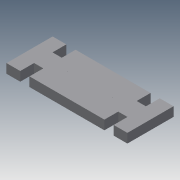
# Autodesk Inventor part: prepazka-sablona
Saved by Autodesk Inventor 2013 (Build 170138000, 138)
## iProperties
Created: 2012-08-25
Part Number: prepazka-sablona
Material: Generic
Document SubType Name: Modeling
Designer: idle-rug
Density: 1 g/cm^3
Author: idle-rug
Autodesk Inventor part; units mm, degrees
ref_plane "YZ Plane" through (0, 0, 0) normal (1, 0, 0) x (0, 1, 0)
ref_plane "XZ Plane" through (0, 0, 0) normal (0, 1, 0) x (-1, 0, 0)
ref_plane "XY Plane" through (0, 0, 0) normal (0, 0, 1) x (1, 0, 0)
sketch "Sketch1" plane through (0, 0, 0) normal (0, 0, 1) x (1, 0, 0)
  line L0 (65.5, 25) -> (-65.5, 25)
  line L1 (-65.5, 25) -> (-65.5, -25)
  line L2 (-65.5, -25) -> (65.5, -25)
  line L3 (65.5, -25) -> (65.5, 25)
  line L4 (-40.6, 25) -> (-40.6, 10)
  line L5 (-40.6, 10) -> (-50.6, 10)
  line L6 (-50.6, 10) -> (-50.6, 25)
  line L7 (-40.6, -25) -> (-40.6, -10)
  line L8 (-40.6, -10) -> (-50.6, -10)
  line L9 (-50.6, -10) -> (-50.6, -25)
  line L10 (40.6, 25) -> (40.6, 10)
  line L11 (40.6, 10) -> (50.6, 10)
  line L12 (50.6, 10) -> (50.6, 25)
  line L13 (40.6, -25) -> (40.6, -10)
  line L14 (40.6, -10) -> (50.6, -10)
  line L15 (50.6, -10) -> (50.6, -25)
  circle A0 centre (-24.1, 0) radius 0.2
  circle A1 centre (24.1, 0) radius 0.2
  point P0 (0, 0)
  point P1 (0, 0)
  dimension "d0" = 15
  dimension "d1" = 15
  dimension "d2" = 15
  dimension "d3" = 15
  dimension "d4" = 0.4
  dimension "d5" = 0.4
  constraints: 32 end point, 8 point on line, 7 perpendicular, 2 centre point
  measures "d0" distance of L4.start L4.end
  measures "d1" distance of L7.start L7.end
  measures "d2" distance of L10.start L10.end
  measures "d3" distance of L13.start L13.end
  measures "d4" diameter of A0
  measures "d5" diameter of A1
extrude "Extrusion1" add sketch "Sketch1" along normal blind 10 contours L3 L2 L15 L14 L13 L7 L8 L9 L1 L0 L6 L5 L4 L10 L11 L12
body "Solid1"
